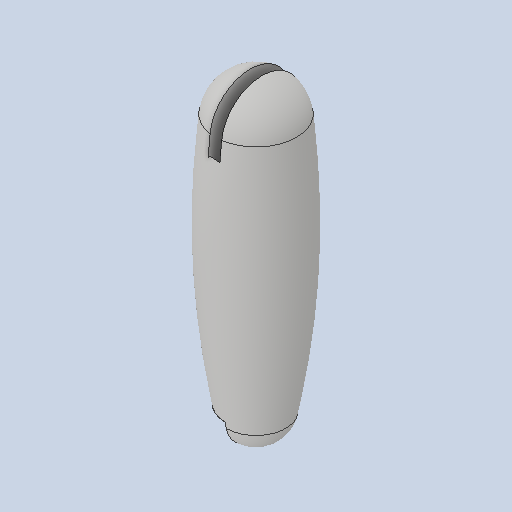
# Autodesk Inventor part: ч ASY human dummy 01
Saved by Autodesk Inventor 2024.2 (Build 282272000, 272)
## iProperties
Created: 2019-08-19
Part Number: ч ASY human dummy 01
Material: Типовые
Document SubType Name: Modeling
Designer: admin
Density: 1 g/cm^3
Appearance: По умолчанию
Author: admin
Autodesk Inventor part; units mm, degrees
ref_plane "YZ Plane" through (0, 0, 0) normal (1, 0, 0) x (0, 1, 0)
ref_plane "XZ Plane" through (0, 0, 0) normal (0, 1, 0) x (-1, 0, 0)
ref_plane "XY Plane" through (0, 0, 0) normal (0, 0, 1) x (1, 0, 0)
sketch "Эскиз1" plane through (0, 0, 0) normal (0, 0, 1) x (1, 0, 0)
  arc A0 (0, -70) -> (0, 70) centre (0, 0) ccw construction
  arc A1 (-51.0516, -434.8862) -> (0, -477) centre (0, -425) ccw
  line L0 (0, 0) -> (0, -425)
  arc A2 (-69.5959, 7.5103) -> (-51.0516, -434.8862) centre (1409.3179, -152.0835) ccw
  line L1 (0, 0) -> (0, 70)
  line L2 (0, -425) -> (0, -477)
  arc A3 (-69.5959, 7.5103) -> (0, -70) centre (0, 0) ccw construction
  arc A4 (0, 70) -> (-69.5959, 7.5103) centre (0, 0) ccw
  arc A5 (0, -373) -> (-51.0516, -434.8862) centre (0, -425) ccw construction
  arc A6 (0, -477) -> (0, -373) centre (0, -425) ccw construction
  dimension "d0" = 140
  dimension "d1" = 104
  dimension "d2" = 425
  dimension "d3" = 1487.5
  constraints: 14 point on circle, 7 centre point, 6 end point, 3 point on line, 2 tangent, 2 vertical, 1 coincident
  measures "d0" diameter of A0
  measures "d1" diameter of A1
  measures "d2" distance of L0.start L0.end
  measures "d3" radius of A2
revolve "Вращение1" add sketch "Эскиз1" angle 360 about axis through (0, 0, 0) along (0, -1, 0)
sketch "Эскиз2" plane through (0, 0, 0) normal (1, 0, 0) x (0, 1, 0)
  arc A0 (7.5103, -69.5959) -> (7.5103, 69.5959) centre (0, 0) ccw projected
  circle A1 centre (0, 0) radius 76
  dimension "d8" = 152
  constraints: 1 centre point, 1 coincident
  measures "d8" diameter of A1
extrude "Выдавливание1" cut sketch "Эскиз2" along normal mid plane 20
sketch "Эскиз3" plane through (0, 0, 0) normal (1, 0, 0) x (0, 1, 0)
  arc A0 (-434.8862, 51.0516) -> (-434.8862, -51.0516) centre (-425, 0) ccw projected
  arc A1 (-425, 52) -> (-425, -52) centre (-425, 0) ccw
  line L0 (-425, -52) -> (-425, 52)
  arc A2 (-425, -52) -> (-425, 52) centre (-425, 0) ccw construction
  point P0 (0, 0)
  constraints: 4 point on circle, 2 centre point, 2 coincident, 2 end point, 1 concentric, 1 midpoint, 1 vertical
revolve "Вращение2" cut sketch "Эскиз3" angle 180 about axis through (0, -425, -52) along (0, 0, -1)
sketch "Эскиз4" plane through (0, 0, 0) normal (0, 0, 1) x (1, 0, 0)
  line L0 (0, -477) -> (0, -434.8862) projected
  arc A0 (-69.5959, 7.5103) -> (-51.0516, -434.8862) centre (1409.3179, -152.0835) ccw projected
  line L1 (0, -477) -> (-53, -477)
  line L2 (-53, -477) -> (-53, -424.6321)
  line L3 (-53, -424.6321) -> (0, -424.6321)
  line L4 (0, -424.6321) -> (0, -477)
  point P0 (0, 0)
  dimension "d10" = 53
  constraints: 8 end point, 2 parallel, 1 horizontal, 1 perpendicular, 1 point on circle
  measures "d10" distance of L0.start L1.end
extrude "Выдавливание2" cut sketch "Эскиз4" along normal through all both and the other way through all
equation "\"d0\" = hip_diam"
equation "\"d1\" = knee_diam"
equation "\"d2\" = femur"
equation "\"d3\" = 3.5 * femur"
equation "\"hip_diam\" = 140"
equation "\"knee_diam\" = 104"
equation "\"femur\" = 425"
